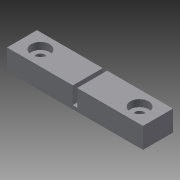
# Autodesk Inventor part: Battery Base
Saved by Autodesk Inventor 2013 (Build 170138000, 138)
## iProperties
Created: 2013-01-15
Part Number: Battery Base
Material: Generic
Document SubType Name: Modeling
Designer: Naphat
Density: 1 g/cm^3
Mass: 25.0675 g
Surface Area: 81.7914 cm^2
Volume: 25.0675 cm^3
Author: Naphat
Autodesk Inventor part; units mm, degrees
ref_plane "YZ Plane" through (0, 0, 0) normal (1, 0, 0) x (0, 1, 0)
ref_plane "XZ Plane" through (0, 0, 0) normal (0, 1, 0) x (-1, 0, 0)
ref_plane "XY Plane" through (0, 0, 0) normal (0, 0, 1) x (1, 0, 0)
sketch "Sketch1" plane through (0, 0, 0) normal (0, 1, 0) x (-1, 0, 0)
  line L0 (85.2904, -33.5134) -> (-8.3721, -33.5134)
  line L1 (-8.3721, -33.5134) -> (-8.3721, -12.8759)
  line L2 (-8.3721, -12.8759) -> (85.2904, -12.8759)
  line L3 (85.2904, -12.8759) -> (85.2904, -33.5134)
  point P0 (0, 0)
  dimension "d0" = 93.6625
  dimension "d1" = 20.6375
  constraints: 8 end point, 2 perpendicular, 1 horizontal, 1 parallel
  measures "d0" distance of L0.start L0.end
  measures "d1" distance of L0.end L1.end
extrude "Extrusion1" add sketch "Sketch1" along normal blind 14.2875
sketch "Sketch2" plane through (0, 14.2875, 0) normal (0, 1, 0) x (1, 0, 0)
  line L0 (8.3721, 33.5134) -> (-85.2904, 33.5134) projected
  line L1 (-85.2904, 33.5134) -> (-85.2904, 12.8759) projected
  line L2 (-85.2904, 12.8759) -> (8.3721, 12.8759) projected
  line L3 (8.3721, 12.8759) -> (8.3721, 33.5134) projected
  line L4 (-85.2904, 23.1947) -> (8.3721, 23.1947) construction
  line L5 (-4.3279, 33.5134) -> (-4.3279, 12.8759) construction
  line L6 (-72.5904, 33.5134) -> (-72.5904, 12.8759) construction
  circle A0 centre (-72.5904, 23.1947) radius 3.175
  circle A1 centre (-4.3279, 23.1947) radius 3.175
  point P0 (0, 0)
  dimension "d4" = 12.7
  dimension "d5" = 12.7
  dimension "d6" = 6.35
  dimension "d7" = 6.35
  constraints: 6 end point, 4 midpoint, 4 point on line, 2 centre point, 1 parallel, 1 perpendicular
  measures "d4" distance between parallel lines of L3 L5
  measures "d5" distance between parallel lines of L1 L6
  measures "d6" diameter of A0
  measures "d7" diameter of A1
extrude "Extrusion2" cut sketch "Sketch2" against normal blind 14.2875 contours A0 | A1
sketch "Sketch3" plane through (0, 14.2875, 0) normal (0, 1, 0) x (1, 0, 0)
  circle A0 centre (-72.5904, 23.1947) radius 3.175 projected
  circle A1 centre (-4.3279, 23.1947) radius 3.175 projected
  circle A2 centre (-72.5904, 23.1947) radius 6.35
  circle A3 centre (-4.3279, 23.1947) radius 6.35
  point P0 (0, 0)
  point P1 (8.3721, 33.5134)
  point P2 (-85.2904, 33.5134)
  dimension "d10" = 12.7
  dimension "d11" = 12.7
  dimension "d14" = 68.2625
  dimension "d16" = 93.6625
  constraints: 2 centre point, 2 coincident
  measures "d10" diameter of A2
  measures "d11" diameter of A3
  measures "d14" distance of A1.centre A0.centre
  measures "d16" distance of point (8.372, 33.513) point (-85.29, 33.513)
extrude "Extrusion3" cut sketch "Sketch3" against normal blind 4.7625
sketch "Sketch4" plane through (0, 14.2875, 0) normal (0, 1, 0) x (1, 0, 0)
  line L0 (8.3721, 33.5134) -> (-85.2904, 33.5134) projected
  line L1 (-85.2904, 12.8759) -> (8.3721, 12.8759) projected
  line L2 (-38.4591, 33.5134) -> (-38.4591, 12.8759) construction
  line L3 (-38.4591, 23.1947) -> (-36.9351, 23.1947) construction
  line L4 (-36.9351, 23.1947) -> (-39.9831, 23.1947) construction
  line L5 (-39.9831, 33.5134) -> (-39.9831, 12.8759)
  line L6 (-39.9831, 12.8759) -> (-36.9351, 12.8759)
  line L7 (-36.9351, 12.8759) -> (-36.9351, 33.5134)
  line L8 (-39.9831, 33.5134) -> (-36.9351, 33.5134)
  point P0 (0, 0)
  dimension "d19" = 1.524
  dimension "d21" = 3.048
  constraints: 14 end point, 5 point on line, 3 midpoint, 3 perpendicular, 1 collinear
  measures "d19" distance of L3.start L3.end
  measures "d21" distance of L3.end L4.end
extrude "Extrusion4" cut sketch "Sketch4" against normal blind 11.7602
equation "\"d5\" = d4"
equation "\"d6\" = d7"
equation "\"d10\" = d11"
body "Solid1"
